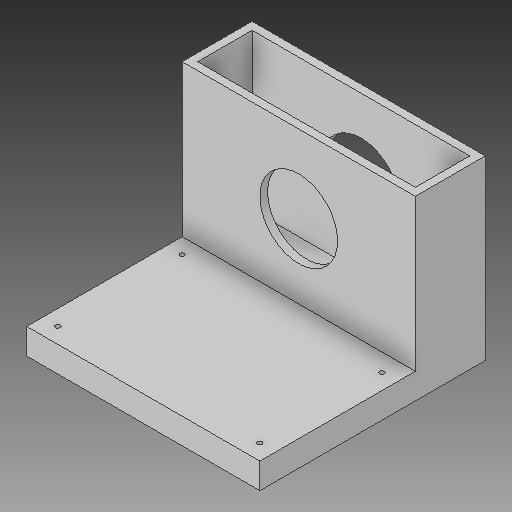
# Autodesk Inventor part: Baseservo
Saved by Autodesk Inventor 2019 (Build 230136000, 136)
## iProperties
Created: 2019-11-21
Part Number: Baseservo
Material: Generic
Document SubType Name: Modeling
Designer: felix
Density: 1 g/cm^3
Appearance: Default
Mass: 4055.19 g
Surface Area: 4821.69 cm^2
Volume: 4055.19 cm^3
Author: felix
Autodesk Inventor part; units mm, degrees
ref_plane "YZ Plane" through (0, 0, 0) normal (1, 0, 0) x (0, 1, 0)
ref_plane "XZ Plane" through (0, 0, 0) normal (0, 1, 0) x (-1, 0, 0)
ref_plane "XY Plane" through (0, 0, 0) normal (0, 0, 1) x (1, 0, 0)
sketch "Sketch1" plane through (0, 0, 0) normal (0, 0, 1) x (1, 0, 0)
  line L0 (0, 0) -> (300, 0)
  line L1 (300, 0) -> (300, 400)
  line L2 (300, 400) -> (0, 400)
  line L3 (0, 400) -> (0, 0)
  dimension "d0" = 300
  dimension "d1" = 400
  constraints: 8 end point, 2 parallel, 1 horizontal, 1 perpendicular
  measures "d0" distance of L2.end L1.end
  measures "d1" distance of L1.end L0.end
extrude "Extrusion1" add sketch "Sketch1" along normal blind 90
sketch "Sketch2" plane through (0, 0, 90) normal (0, 0, 1) x (1, 0, 0)
  circle A0 centre (150, 300) radius 50
  point P0 (0, 0)
  dimension "d4" = 100
  dimension "d5" = 150
  dimension "d6" = 300
  constraints: 1 centre point
  measures "d4" diameter of A0
  measures "d5" horizontal distance of point (0, 0) A0.centre
  measures "d6" vertical distance of point (0, 0) A0.centre
extrude "Extrusion2" cut sketch "Sketch2" against normal blind 100
sketch "Sketch4" plane through (0, 400, 0) normal (0, 1, 0) x (1, 0, 0)
  line L0 (10, -80) -> (290, -80)
  line L1 (290, -80) -> (290, -10)
  line L2 (290, -10) -> (10, -10)
  line L3 (10, -10) -> (10, -80)
  line L4 (0, 0) -> (0, -90) projected
  dimension "d12" = 70
  dimension "d13" = 280
  dimension "d14" = 10
  dimension "d15" = 10
  constraints: 8 end point, 2 parallel, 1 horizontal, 1 perpendicular
  measures "d12" distance of L2.end L0.start
  measures "d13" distance of L1.end L2.end
  measures "d14" distance from line of L4 L2.end
  measures "d15" distance from line of L2 L4.start
extrude "Extrusion4" cut sketch "Sketch4" against normal blind 200
sketch "Sketch5" plane through (0, 0, 90) normal (0, 0, 1) x (1, 0, 0)
  line L0 (0, 205) -> (300, 205)
  line L1 (300, 400) -> (0, 400) projected
  line L2 (0, 400) -> (0, 0) projected
  line L3 (300, 0) -> (300, 400) projected
  line L4 (0, 205) -> (0, 172)
  line L5 (0, 172) -> (300, 172)
  line L6 (300, 0) -> (300, 400) projected
  line L7 (300, 205) -> (300, 172)
  dimension "d18" = 195
  dimension "d19" = 33
  constraints: 8 end point, 4 point on line, 1 collinear, 1 horizontal, 1 perpendicular
  measures "d18" distance between parallel lines of L0 L1
  measures "d19" distance of L0.start L4.end
extrude "Extrusion5" add sketch "Sketch5" along normal blind 200 contours L0 L3 L5 L2
sketch "Sketch6" plane through (0, 0, 0) normal (0, -1, 0) x (1, 0, 0)
  line L0 (300, 90) -> (0, 90) projected
  line L1 (0, 0) -> (300, 0)
  line L2 (300, 0) -> (300, 90)
  line L3 (300, 90) -> (0, 90)
  line L4 (0, 90) -> (0, 0)
  constraints: 8 end point, 2 parallel, 1 horizontal, 1 perpendicular
extrude "Extrusion6" cut sketch "Sketch6" against normal blind 172
sketch "Sketch7" plane through (0, 205, 90) normal (0, 1, 0) x (1, 0, 0)
  circle A0 centre (20, -180) radius 3
  circle A1 centre (20, -20) radius 3
  circle A2 centre (280, -23) radius 3
  circle A3 centre (280, -180) radius 3
  line L0 (300, -200) -> (0, -200) projected
  line L1 (0, 0) -> (0, -200) projected
  line L2 (300, 0) -> (0, 0) projected
  line L3 (300, 0) -> (300, -200) projected
  point P0 (0, 90)
  dimension "d24" = 20
  dimension "d25" = 20
  dimension "d26" = 6
  dimension "d27" = 20
  dimension "d28" = 20
  dimension "d29" = 20
  dimension "d30" = 20
  dimension "d31" = 20
  dimension "d32" = 20
  constraints: 4 centre point, 3 equal radius
  measures "d24" distance from line of A0.centre L0
  measures "d25" distance from line of L1 A0.centre
  measures "d26" diameter of A0
  measures "d27" distance from line of L2 A1.centre
  measures "d28" distance from line of L1 A1.centre
  measures "d29" distance edge to line of A2 L2
  measures "d30" distance from line of L3 A2.centre
  measures "d31" distance from line of L0 A3.centre
  measures "d32" distance from line of L3 A3.centre
extrude "Extrusion7" cut sketch "Sketch7" against normal blind 50 contours A0 | A1 | A2 | A3
body "Solid1"
